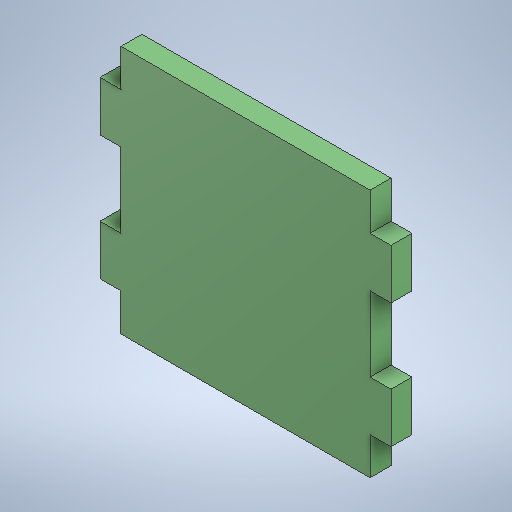
# Autodesk Inventor part: 7
Saved by Autodesk Inventor 2025.3 (Build 293356000, 356)
## iProperties
Created: 2025-12-22
Part Number: 7
Material: Generic
Document SubType Name: Sheet Metal
Designer: Balint
Density: 1 g/cm^3
Sheet Metal Rule: Default_mm
Appearance: Default
Flat Pattern Width: 21.4 cm
Flat Pattern Length: 25 cm
Flat Pattern Area: 535 cm^2
Sheet Metal Width: 214.000 mm
Sheet Metal Length: 250.000 mm
Sheet Metal Area: 53500.000 mm^2
Author: Balint
Autodesk Inventor part; units mm, degrees
ref_plane "YZ Plane" through (0, 0, 0) normal (1, 0, 0) x (0, 1, 0)
ref_plane "XZ Plane" through (0, 0, 0) normal (0, 1, 0) x (-1, 0, 0)
ref_plane "XY Plane" through (0, 0, 0) normal (0, 0, 1) x (1, 0, 0)
sketch "Sketch1" plane through (0, 0, 0) normal (0, 0, 1) x (1, 0, 0)
  line L0 (232, 157.1) -> (-18, 157.1)
  line L1 (-18, 157.1) -> (-18, -92.9)
  line L2 (-18, -92.9) -> (232, -92.9)
  line L3 (232, -92.9) -> (232, 157.1)
  line L4 (-18, -42.8) -> (0, -42.8)
  line L5 (0, -42.8) -> (0, -92.9)
  line L6 (0, -92.9) -> (-18, -92.9)
  line L7 (-18, -92.9) -> (-18, -42.8)
  line L8 (0, 107) -> (0, 64.2)
  line L9 (0, 64.2) -> (-18, 64.2)
  line L10 (-18, 64.2) -> (-18, 107)
  line L11 (76.5522, 157.3937) -> (94.5522, 157.3937)
  line L12 (-18, -42.8) -> (-18, 0)
  line L13 (-18, 0) -> (0, 0)
  line L14 (0, 0) -> (0, -42.8)
  line L15 (0, -42.8) -> (-18, -42.8)
  line L16 (-18, -42.8) -> (0, -42.8)
  line L17 (0, -42.8) -> (0, 0)
  line L18 (0, 0) -> (-18, 0)
  line L19 (-18, 0) -> (-18, -42.8)
  line L20 (0, 0) -> (-18, 0)
  line L21 (-18, 0) -> (-18, 64.2)
  line L22 (-18, 64.2) -> (0, 64.2)
  line L23 (0, 64.2) -> (0, 0)
  line L24 (-18, 64.2) -> (-18, 107)
  line L25 (0, 64.2) -> (-18, 64.2)
  line L26 (-18, 64.2) -> (-18, 107)
  line L27 (76.5522, 157.3937) -> (94.5522, 157.3937)
  line L28 (0, 107) -> (0, 64.2)
  line L29 (76.5522, 157.3937) -> (94.5522, 157.3937)
  line L30 (0, 107) -> (0, 157.1)
  line L31 (0, 157.1) -> (-18, 157.1)
  line L32 (-18, 157.1) -> (-18, 107)
  line L33 (0, 64.2) -> (0, 107)
  line L34 (0, 107) -> (-18, 107)
  line L35 (232, -92.9) -> (94.5522, -92.9)
  line L36 (-18, -92.9) -> (107, -92.9)
  line L37 (107, -92.9) -> (107, 52.5886)
  line L38 (232, 157.1) -> (232, -92.9)
  line L39 (232, -42.8) -> (214, -42.8)
  line L40 (232, -92.9) -> (232, -42.8)
  line L41 (214, -42.8) -> (214, -92.9)
  line L42 (214, 107) -> (214, 64.2)
  line L43 (214, 107) -> (214, 64.2)
  line L44 (232, 64.2) -> (232, 107)
  line L45 (232, 64.2) -> (232, 107)
  line L46 (232, 64.2) -> (232, 107)
  line L47 (214, 107) -> (214, 157.1)
  line L48 (232, 157.1) -> (232, 107)
  line L49 (214, -42.8) -> (232, -42.8)
  line L50 (232, -42.8) -> (214, -42.8)
  line L51 (214, -42.8) -> (214, 0)
  line L52 (232, -42.8) -> (232, 0)
  line L53 (232, 0) -> (214, 0)
  line L54 (232, 0) -> (232, -42.8)
  line L55 (214, 0) -> (232, 0)
  line L56 (214, 0) -> (232, 0)
  line L57 (214, 64.2) -> (214, 0)
  line L58 (214, 64.2) -> (232, 64.2)
  line L59 (232, 0) -> (232, 64.2)
  line L60 (214, 64.2) -> (232, 64.2)
  line L61 (232, 64.2) -> (214, 64.2)
  line L62 (214, 0) -> (214, -42.8)
  line L63 (214, 64.2) -> (214, 107)
  line L64 (214, 107) -> (232, 107)
  line L65 (214, 157.1) -> (0, 157.1)
  line L66 (0, 157.1) -> (0, 139.1)
  line L67 (0, 139.1) -> (214, 139.1)
  line L68 (214, 139.1) -> (214, 157.1)
  line L69 (232, 157.1) -> (-18, 157.1)
  line L70 (-18, 157.1) -> (-18, 139.1)
  line L71 (-18, 139.1) -> (232, 139.1)
  line L72 (232, 139.1) -> (232, 157.1)
  line L73 (232, -92.9) -> (-18, -92.9)
  line L74 (-18, -92.9) -> (-18, -74.9)
  line L75 (-18, -74.9) -> (232, -74.9)
  line L76 (232, -74.9) -> (232, -92.9)
  point P0 (0, 0)
  point P1 (214, 0)
  point P2 (0, -74.9)
  point P3 (214, -74.9)
  dimension "d0" = 18
  dimension "d1" = 42.8
  dimension "d2" = 125
  dimension "d4" = 18
  dimension "d5" = 18
  measures "d0" distance of L6.start L7.start
  measures "d1" distance of L28.end L33.end
  measures "d2" distance of L7.start L36.end
  measures "d4" distance of L66.end L65.end
  measures "d5" distance of L73.end L74.end
extrude "Plate1" add sketch "Sketch1" along normal blind 18 contours L47 L42 L57 L51 L41 L75 L5 L14 L23 L8 L30 L67 | L3 L58 L42 L64 | L8 L9 L1 L34 | L3 L39 L51 L53 | L14 L4 L1 L13
equation "\"d3\" = Thickness"
equation "\"BendRadius\" = Thickness"
equation "\"BendReliefWidth\" = Thickness"
equation "\"BendReliefDepth\" = 0.5 * Thickness"
equation "\"CornerReliefSize\" = 4 * Thickness"
equation "\"MinimumRemnant\" = 2 * Thickness"
equation "\"TransitionRadius\" = BendRadius"
equation "\"JacobiRadiusSize\" = BendRadius"
equation "\"GapSize\" = Thickness"
equation "\"Thickness\" = 18"
body "Solid1"
